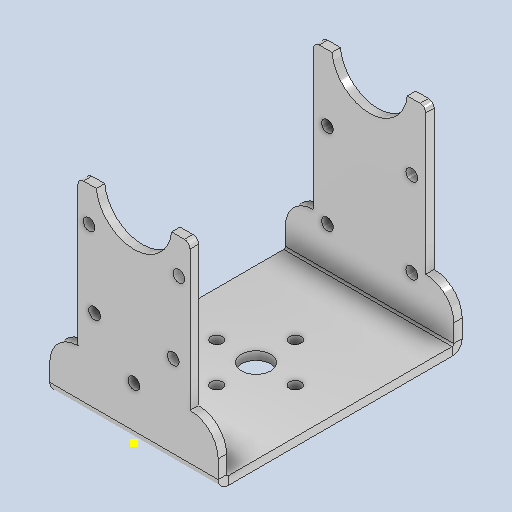
# Autodesk Inventor part: axis_19_top_frame
Saved by Autodesk Inventor 2026.1 (Build 301233020, 233B)
## iProperties
Created: 2025-05-06
Part Number: axis_19_top_frame
Material: Aluminum 6061-AHC
Document SubType Name: Sheet Metal
Designer: LG
Density: 2.7 g/cm^3
Sheet Metal Rule: Default_mm
Appearance: Aluminum - Dark
Author: LG
Autodesk Inventor part; units mm, degrees
ref_plane "YZ Plane" through (0, 0, 0) normal (1, 0, 0) x (0, 1, 0)
ref_plane "XZ Plane" through (0, 0, 0) normal (0, 1, 0) x (-1, 0, 0)
ref_plane "XY Plane" through (0, 0, 0) normal (0, 0, 1) x (1, 0, 0)
sketch "Sketch1" plane through (0, 0, 0) normal (0, 1, 0) x (-1, 0, 0)
  line L0 (-15, 20.25) -> (15, 20.25)
  line L1 (15, 20.25) -> (15, -20.25)
  line L2 (15, -20.25) -> (-15, -20.25)
  line L3 (-15, -20.25) -> (-15, 20.25)
  line L4 (-15, 20.25) -> (15, -20.25) construction
  line L5 (15, 20.25) -> (-15, -20.25) construction
  point P0 (0, 0)
  dimension "d0" = 40.5
  dimension "d1" = 30
  measures "d0" distance of L0.end L1.end
  measures "d1" distance of L1.end L2.end
extrude "Plate1" add sketch "Sketch1" along normal blind 1.5
sketch "Sketch2" plane through (-15, 0, -21.75) normal (0, 0, 1) x (1, 0, 0)
  line L0 (30, 0) -> (0, 0)
  line L1 (0, 0) -> (0, 35.9)
  line L2 (0, 35.9) -> (30, 35.9)
  line L3 (30, 35.9) -> (30, 0)
  constraints: 8 end point
edge flange "Flange1" height 35.9 angle 90 thickness 1.5 bend radius 0.31 thickness toward (0, 0, 1) relief tear relief width 1.5 relief depth 0.75 corner gap 0.31 corner form 0 edges at (0, 1.5, -20.25) (0, 1.5, 20.25) wall of the first edge with corners at (15, 0, -21.75) (-15, 0, -21.75) (-15, 35.9, -21.75) (15, 35.9, -21.75)
bend "Bend1"
corner "Corner1"
sketch "Sketch3" plane through (0, 1.5, 0) normal (0, 1, 0) x (1, 0, 0)
  circle A0 centre (7, 0) radius 0.7835 projected
  circle A1 centre (0, -7) radius 0.7835 projected
  circle A2 centre (-7, 0) radius 0.7835 projected
  circle A3 centre (0, 7) radius 0.7835 projected
  point P0 (0, 0)
hole "Hole1" at (0, 1.5, 7) at (7, 1.5, 0) at (-7, 1.5, 0) at (0, 1.5, -7) direction (0, -1, 0) diameter 2.1 depth 1.5
sketch "Sketch26" plane through (-15, 35.9, 21.75) normal (0, 0, 1) x (1, 0, 0)
  line L0 (30, 9.1) -> (25, 9.1)
  line L1 (25, 9.1) -> (25, -25.9)
  line L2 (25, -25.9) -> (30, -25.9)
  line L3 (30, -25.9) -> (30, 9.1)
  line L4 (0, 9.1) -> (5, 9.1)
  line L5 (5, 9.1) -> (5, -25.9)
  line L6 (5, -25.9) -> (0, -25.9)
  line L7 (0, -25.9) -> (0, 9.1)
  point P0 (15, -35.9)
  dimension "d91" = 35
  dimension "d92" = 5
  dimension "d93" = 10
  dimension "d94" = 10
  dimension "d95" = 5
  dimension "d96" = 35
  dimension "d97" = 10
  dimension "d98" = 10
  constraints: 16 end point, 4 parallel, 2 horizontal, 2 perpendicular
  measures "d91" distance of L2.end L0.start
  measures "d92" distance of L1.end L2.end
  measures "d93" distance from line of point (15, -35.9) L1
  measures "d94" distance from line of point (15, -35.9) L2
  measures "d95" distance of L5.end L6.end
  measures "d96" distance of L4.end L5.end
  measures "d97" distance from line of point (15, -35.9) L6
  measures "d98" distance from line of point (15, -35.9) L5
extrude "Cut11" cut sketch "Sketch26" against normal blind 1.5
fillet "Corner Round1" radius 5 1 edges at (-15, 10, 21)
fillet "Corner Round2" radius 5 1 edges at (15, 10, 21)
mirror "Mirror1" about plane through (0, 0, 0) normal (0, 0, 1) of "Cut11"
fillet "Corner Round3" radius 5 1 edges at (-15, 10, -21)
fillet "Corner Round4" radius 5 1 edges at (15, 10, -21)
fillet "Corner Round5" radius 1 4 edges at (10, 35.9, -21) (10, 35.9, 21) (-10, 35.9, 21) (-10, 35.9, -21)
sketch "Sketch31" plane through (-15, 1.81, 21.75) normal (0, 0, 1) x (1, 0, 0)
  point P0 (15, -1.81)
sketch "Sketch34" plane through (0, 1.5, 0) normal (0, 1, 0) x (1, 0, 0)
  circle A0 centre (0, 0) radius 1.2295
  point P0 (0, 0)
  constraints: 1 centre point, 2 other
hole "Hole13" at (0, 1.5, 0) direction (0, -1, 0) diameter 5.2 depth 1.5
sketch "Sketch35" plane through (-15, 1.81, 21.75) normal (0, 0, 1) x (1, 0, 0)
  circle A0 centre (15, 34.79) radius 2.925
  point P0 (15, -1.81)
  constraints: 1 centre point, 2 other
hole "Hole16" at (0, 36.6, 21.75) direction (0, 0, -1) diameter 13.5 depth 1.5
sketch "Sketch36" plane through (15, 1.81, -21.75) normal (0, 0, -1) x (-1, 0, 0)
  circle A0 centre (15, 34.79) radius 4.48
  point P0 (15, -1.81)
  constraints: 1 centre point, 2 other
hole "Hole17" at (0, 36.6, -21.75) direction (0, 0, 1) diameter 13.5 depth 1.5
sketch "Sketch37" plane through (-15, 1.81, 21.75) normal (0, 0, 1) x (1, 0, 0)
  circle A0 centre (23, 27.89) radius 0.7835
  circle A1 centre (22, 14.67) radius 0.7835
  circle A2 centre (15, 7.37) radius 0.7835
  circle A3 centre (8, 14.67) radius 0.7835
  circle A4 centre (7, 27.89) radius 0.7835
  point P0 (15, -1.81)
  constraints: 5 centre point, 10 other
hole "Hole18" at (8, 29.7, 21.75) at (-8, 29.7, 21.75) at (7, 16.48, 21.75) at (-7, 16.48, 21.75) at (0, 9.18, 21.75) direction (0, 0, -1) diameter 2.1 depth 1.5
sketch "Sketch38" plane through (15, 1.81, -21.75) normal (0, 0, -1) x (-1, 0, 0)
  circle A0 centre (7.475, 7.19) radius 0.7835
  circle A1 centre (7.475, 22.29) radius 0.7835
  circle A2 centre (22.525, 7.19) radius 0.7835
  circle A3 centre (22.525, 22.29) radius 0.7835
  point P0 (15, -1.81)
  constraints: 4 centre point, 8 other
hole "Hole19" at (7.525, 9, -21.75) at (7.525, 24.1, -21.75) at (-7.525, 9, -21.75) at (-7.525, 24.1, -21.75) direction (0, 0, 1) diameter 2.1 depth 1.5
equation "\"d18\" = Thickness"
equation "\"d99\" = Thickness"
equation "\"d143\" = Thickness"
equation "\"d164\" = Thickness"
equation "\"d171\" = Thickness"
equation "\"d178\" = Thickness"
equation "\"d185\" = Thickness"
equation "\"d2\" = Thickness"
equation "\"d3\" = BendReliefWidth"
equation "\"d4\" = BendReliefDepth"
equation "\"d5\" = MinimumRemnant"
equation "\"d6\" = TransitionRadius"
equation "\"d9\" = BendRadius"
equation "\"d10\" = CornerReliefSize"
equation "\"d11\" = GapSize"
equation "\"d12\" = JacobiRadiusSize"
equation "\"BendReliefWidth\" = Thickness"
equation "\"BendReliefDepth\" = 0.5 * Thickness"
equation "\"CornerReliefSize\" = 4 * Thickness"
equation "\"MinimumRemnant\" = 2 * Thickness"
equation "\"TransitionRadius\" = BendRadius"
equation "\"JacobiRadiusSize\" = BendRadius"
equation "\"GapSize\" = Thickness"
equation "\"Thickness\" = 1.5"
equation "\"BendRadius\" = 0.31"
body "Solid1"
